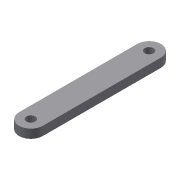
# Autodesk Inventor part: bar1
Saved by Autodesk Inventor 2018 (Build 220112000, 112)
## iProperties
Created: 2018-05-25
Part Number: bar1
Material: Generic
Document SubType Name: Modeling
Designer: Bardo91
Density: 1 g/cm^3
Appearance: Default
Author: Bardo91
Autodesk Inventor part; units mm, degrees
ref_plane "YZ Plane" through (0, 0, 0) normal (1, 0, 0) x (0, 1, 0)
ref_plane "XZ Plane" through (0, 0, 0) normal (0, 1, 0) x (-1, 0, 0)
ref_plane "XY Plane" through (0, 0, 0) normal (0, 0, 1) x (1, 0, 0)
sketch "Sketch1" plane through (0, 0, 0) normal (0, 0, 1) x (1, 0, 0)
  circle A0 centre (0, 0) radius 1.5
  circle A1 centre (0, 0) radius 4
  line L0 (0, 0) -> (0, 40)
  circle A2 centre (0, 40) radius 1.5
  circle A3 centre (0, 40) radius 4
  line L1 (-4, 40) -> (-4, 0)
  line L2 (4, 40) -> (4, 0)
  dimension "d0" = 3
  dimension "d1" = 8
  dimension "d2" = 40
  dimension "d3" = 3
  dimension "d4" = 8
  constraints: 6 end point, 4 centre point, 4 coincident, 4 point on circle, 2 vertical, 1 parallel, 1 tangent
  measures "d0" diameter of A0
  measures "d1" diameter of A1
  measures "d2" distance of L0.start L0.end
  measures "d3" diameter of A2
  measures "d4" diameter of A3
extrude "Extrusion1" add sketch "Sketch1" along normal blind 3
body "Solid1"
